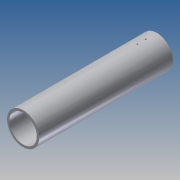
# Autodesk Inventor part: 2h2slv
Saved by Autodesk Inventor 2014 SP1 (Build 180222100, 222)
## iProperties
Company: HERA Project
Created: 2013-05-14
Part Number: 2h2slv
Material: PVC-Piping
Document SubType Name: Modeling
Designer: David DeBoer
Density: 1.4 g/cm^3
Mass: 429.807 g
Surface Area: 1214.86 cm^2
Volume: 307.005 cm^3
Description: Hub mating sleeve
Appearance: Smooth - White
Author: David DeBoer
Title: Hub mating sleeve
Autodesk Inventor part; units mm, degrees
ref_plane "YZ Plane" through (0, 0, 0) normal (1, 0, 0) x (0, 1, 0)
sketch "Sketch1" plane through (0, 0, 0) normal (0, 0, 1) x (1, 0, 0)
  circle A0 centre (0, 0) radius 36.5125
  circle A1 centre (0, 0) radius 31.3563
  dimension "d0" = 73.025
  dimension "d2" = 5.1562
  constraints: 2 centre point, 1 coincident
  measures "d0" diameter of A0
  measures "d2" radial gap between concentric circles of A1 A0
extrude "Extrusion1" add sketch "Sketch1" along normal blind 304.8
sketch "Sketch2" plane through (0, 0, 304.8) normal (0, 0, 1) x (1, 0, 0)
  circle A0 centre (0, 0) radius 31.3563 projected
  circle A1 centre (0, 0) radius 36.5125 projected
  point P0 (0, 36.5125)
  constraints: 1 vertical alignment, 1 other
ref_plane "Work Plane1" through (0, 36.5125, 304.8) normal (0, 1, 0) x (-1, 0, 0)
sketch "Sketch5" plane through (0, 36.5125, 304.8) normal (0, 1, 0) x (-1, 0, 0)
  circle A0 centre (0, -279.4) radius 4.4901
  circle A1 centre (0, -260.35) radius 4.4901
  point P0 (0, -304.8)
  dimension "d25" = 25.4
  dimension "d26" = 19.05
  constraints: 2 centre point
  measures "d25" distance of point (0, -304.8) A0.centre
  measures "d26" distance of A0.centre A1.centre
hole "Hole3" at (0, 36.5125, 44.45) at (0, 36.5125, 25.4) direction (0, -1, 0) diameter 3.175 end through all
sketch "Sketch6" plane through (0, 0, 304.8) normal (0, 0, 1) x (1, 0, 0)
  circle A0 centre (0, 0) radius 31.3563 projected
  circle A1 centre (0, 0) radius 36.5125 projected
  point P0 (0, 36.5125)
  constraints: 1 vertical alignment, 1 other
ref_plane "Work Plane2" through (0, 36.5125, 304.8) normal (0, 1, 0) x (-1, 0, 0)
sketch "Sketch9" plane through (0, 0, 304.8) normal (0, 0, 1) x (1, 0, 0)
  circle A0 centre (0, 0) radius 31.3563 projected
  circle A1 centre (0, 0) radius 36.5125 projected
  line L0 (-1.27, 30.7627) -> (1.27, 30.7627)
  line L1 (1.27, 30.7627) -> (1.27, 33.3027)
  line L2 (1.27, 33.3027) -> (-1.27, 33.3027)
  line L3 (-1.27, 33.3027) -> (-1.27, 30.7627)
  line L4 (0, 33.3027) -> (0, 30.7627) construction
  line L5 (0, 31.3563) -> (0, 36.5125) construction
  dimension "d38" = 2.54
  dimension "d39" = 2.54
  constraints: 12 end point, 2 collinear, 2 midpoint, 2 parallel, 2 vertical alignment, 1 horizontal, 1 perpendicular, 2 other
  measures "d38" distance of L2.end L1.end
  measures "d39" distance of L1.end L0.end
extrude "Extrusion3" cut sketch "Sketch9" against normal blind 25.4 contours L1 L0 L3 A0 | A0 L3 L2 L1 picked at (0.1411, 30.9596)
body "Solid1"
